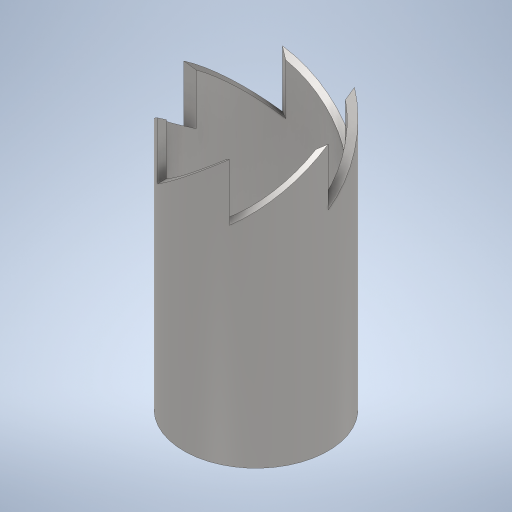
# Autodesk Inventor part: sheller
Saved by Autodesk Inventor 2024.2 (Build 282272000, 272)
## iProperties
Created: 2024-05-25
Part Number: sheller
Material: Stainless Steel
Document SubType Name: Modeling
Designer: user
Density: 8 g/cm^3
Appearance: Semi-Polished
Author: user
Autodesk Inventor part; units mm, degrees
ref_plane "YZ Plane" through (0, 0, 0) normal (1, 0, 0) x (0, 1, 0)
sketch "Sketch1" plane through (0, 0, 0) normal (0, 1, 0) x (-1, 0, 0)
  circle A0 centre (0, 0) radius 19
  dimension "d0" = 38
  constraints: 1 centre point, 1 coincident
  measures "d0" diameter of A0
extrude "Extrusion1" add sketch "Sketch1" along normal blind 70
ref_plane "Work Plane1" through (0, 70, 0) normal (0, 1, 0) x (-1, 0, 0)
sketch "Sketch2" plane through (0, 70, 0) normal (0, 1, 0) x (-1, 0, 0)
  line L0 (0, 0) -> (9.5, -16.4545)
  circle A0 centre (0, 0) radius 19 projected
  line L1 (26.6, 0) -> (-26.6, 0) projected
  point P0 (19, 0)
  point P1 (9.5, 16.4545)
  point P2 (-9.5, 16.4545)
  point P3 (-19, 0)
  point P4 (-9.5, -16.4545)
  dimension "d4" = 60
  dimension "d7" = 360
  constraints: 2 end point, 1 coincident, 9 other
  measures "d4" angle of L0 L1
ref_plane "Work Plane2" through (0, 0, 19) normal (0, 0, 1) x (1, 0, 0)
sketch "Sketch3" plane through (0, 0, 19) normal (0, 0, 1) x (1, 0, 0)
  line L0 (19, 70) -> (-19, 70) projected
  line L1 (19, 55) -> (-19, 55)
  line L2 (-9.5, 70) -> (-9.5, 55)
  line L3 (9.5, 70) -> (-9.5, 55)
  line L4 (-9.5, 70) -> (9.5, 70)
  line L5 (19, 70) -> (-19, 70) projected
  point P0 (0, 0)
  dimension "d10" = 15
  constraints: 8 end point, 1 collinear, 1 parallel, 1 perpendicular, 1 point on line
  measures "d10" distance between parallel lines of L0 L1
extrude "Extrusion2" cut sketch "Sketch3" against normal up to surface (19 mm away)
pattern_circular "Circular Pattern1" count 6 over 360 about axis through (0, -10, 0) along (0, 1, 0) of "Extrusion2"
shell "Shell1" thickness 2 removed faces 19 at (-4.7406, 0, -4.1998) at (11.0833, 56.25, 2.7424) at (-3.1667, 56.25, -10.9697) at (3.1667, 56.25, 10.9697) at (4.75, 58.75, -2.7424) at (-3.1667, 58.75, 5.4848) at (-11.0833, 56.25, -2.7424) at (-7.9167, 56.25, 8.2272) at (-9.5, 61.25, 10.9697) at (4.75, 61.25, 13.7121) at (9.5, 61.25, -10.9697) at (6.3333, 58.75, 0) at (3.1667, 58.75, -5.4848) at (-4.75, 61.25, -13.7121) at (-14.25, 61.25, -2.7424) at (-6.3333, 58.75, 0) at (3.1667, 58.75, 5.4848) at (14.25, 61.25, 2.7424) at (-3.1667, 58.75, -5.4848)
body "Solid1"
